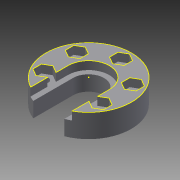
# Autodesk Inventor part: Kossel E3D V6 Mount
Saved by Autodesk Inventor 2013 (Build 170138000, 138)
## iProperties
Created: 2014-06-22
Part Number: Kossel E3D V6 Mount
Material: Generic
Document SubType Name: Modeling
Designer: Enlightx
Density: 1 g/cm^3
Author: Enlightx
Autodesk Inventor part; units mm, degrees
ref_plane "YZ Plane" through (0, 0, 0) normal (1, 0, 0) x (0, 1, 0)
ref_plane "XZ Plane" through (0, 0, 0) normal (0, 1, 0) x (-1, 0, 0)
ref_plane "XY Plane" through (0, 0, 0) normal (0, 0, 1) x (1, 0, 0)
sketch "Sketch1" plane through (0, 0, 0) normal (0, 0, 1) x (1, 0, 0)
  circle A0 centre (0, 0) radius 16.5
  dimension "d0" = 33
  constraints: 1 centre point, 1 coincident
  measures "d0" diameter of A0
extrude "Body" add sketch "Sketch1" along normal blind 9
sketch "Sketch2" plane through (0, 0, 9) normal (0, 0, 1) x (1, 0, 0)
  circle A0 centre (0, 0) radius 16.5 projected
  circle A1 centre (0, 0) radius 6
  line L0 (-6, 0) -> (-6, -15.3704)
  line L1 (6, 0) -> (6, -15.3704)
  arc A2 (-6, -15.3704) -> (6, -15.3704) centre (0, 0) ccw
  dimension "d3" = 12
  constraints: 6 point on circle, 4 end point, 2 centre point, 2 tangent, 1 coincident, 1 concentric, 1 parallel, 1 vertical
  measures "d3" diameter of A1
extrude "Main Cutout" cut sketch "Sketch2" against normal blind 9 contours L0 A1 L1 A0 | A1 picked at (0.2411, -12.9009)
sketch "Sketch4" plane through (0, 0, 9) normal (0, 0, 1) x (1, 0, 0)
  line L0 (6, 0) -> (6, -15.3704) projected
  arc A0 (6, -15.3704) -> (-6, -15.3704) centre (0, 0) ccw projected
  line L1 (-6, -15.3704) -> (-6, 0) projected
  arc A1 (6, 0) -> (-6, 0) centre (0, 0) ccw projected
  circle A2 centre (0, 0) radius 8
  line L2 (-8, 0) -> (-8, -14.4309)
  line L3 (8, 0) -> (8, -14.4309)
  arc A3 (-8, -14.4309) -> (8, -14.4309) centre (0, 0) ccw
  dimension "d7" = 16
  constraints: 6 point on circle, 4 end point, 2 centre point, 2 parallel, 2 tangent, 1 coincident, 1 concentric
  measures "d7" diameter of A2
extrude "Bottom Cutout" cut sketch "Sketch4" against normal blind 3.2 contours A1 L1 A2 L0 | A2 L3 A0 L0 | L1 A0 L2 A2 picked at (-6.3631, -2.9996)
sketch "Sketch7" plane through (0, 0, 0) normal (0, 0, -1) x (-1, 0, 0)
  arc A0 (6, 0) -> (-6, 0) centre (0, 0) ccw projected
  arc A1 (6, -15.3704) -> (-6, -15.3704) centre (0, 0) ccw projected
  circle A2 centre (0, 0) radius 12.5 construction
  circle A3 centre (0, 12.5) radius 1.6
  circle A4 centre (-10.8253, 6.25) radius 1.6
  circle A5 centre (-10.8253, -6.25) radius 1.6
  circle A6 centre (0, -12.5) radius 1.6
  circle A7 centre (10.8253, -6.25) radius 1.6
  circle A8 centre (10.8253, 6.25) radius 1.6
  dimension "d18" = 25
  dimension "d19" = 3.2
  dimension "d22" = 360
  constraints: 6 centre point, 1 coincident, 1 vertical alignment, 15 other
  measures "d19" diameter of A3
extrude "M3 Holes" cut sketch "Sketch7" against normal blind 7 contours A3 | A4 | A5 | A7 | A8
sketch "Sketch8" plane through (0, 0, 9) normal (0, 0, 1) x (1, 0, 0)
  arc A0 (8, 0) -> (-8, 0) centre (0, 0) ccw projected
  circle A1 centre (0, 0) radius 12.5 construction
  circle A2 centre (0, 12.5) radius 1.5 construction
  circle A3 centre (-10.8253, 6.25) radius 1.5 construction
  circle A4 centre (-10.8253, -6.25) radius 1.5 construction
  circle A5 centre (0, -12.5) radius 1.5 construction
  circle A6 centre (10.8253, -6.25) radius 1.5 construction
  circle A7 centre (10.8253, 6.25) radius 1.5 construction
  line L0 (0, 9.238) -> (-2.825, 10.869)
  line L1 (-2.825, 10.869) -> (-2.825, 14.131)
  line L2 (-2.825, 14.131) -> (0, 15.762)
  line L3 (0, 15.762) -> (2.825, 14.131)
  line L4 (2.825, 14.131) -> (2.825, 10.869)
  line L5 (2.825, 10.869) -> (0, 9.238)
  line L6 (-10.8253, 2.988) -> (-13.6503, 4.619)
  line L7 (-13.6503, 4.619) -> (-13.6503, 7.881)
  line L8 (-13.6503, 7.881) -> (-10.8253, 9.512)
  line L9 (-10.8253, 9.512) -> (-8.0003, 7.881)
  line L10 (-8.0003, 7.881) -> (-8.0003, 4.619)
  line L11 (-8.0003, 4.619) -> (-10.8253, 2.988)
  line L12 (10.8253, 2.988) -> (8.0003, 4.619)
  line L13 (8.0003, 4.619) -> (8.0003, 7.881)
  line L14 (8.0003, 7.881) -> (10.8253, 9.512)
  line L15 (10.8253, 9.512) -> (13.6503, 7.881)
  line L16 (13.6503, 7.881) -> (13.6503, 4.619)
  line L17 (13.6503, 4.619) -> (10.8253, 2.988)
  line L18 (-10.8253, -9.5178) -> (-13.6553, -7.8839)
  line L19 (-13.6553, -7.8839) -> (-13.6553, -4.6161)
  line L20 (-13.6553, -4.6161) -> (-10.8253, -2.9822)
  line L21 (-10.8253, -2.9822) -> (-7.9953, -4.6161)
  line L22 (-7.9953, -4.6161) -> (-7.9953, -7.8839)
  line L23 (-7.9953, -7.8839) -> (-10.8253, -9.5178)
  line L24 (10.8253, -9.5178) -> (7.9953, -7.8839)
  line L25 (7.9953, -7.8839) -> (7.9953, -4.6161)
  line L26 (7.9953, -4.6161) -> (10.8253, -2.9822)
  line L27 (10.8253, -2.9822) -> (13.6553, -4.6161)
  line L28 (13.6553, -4.6161) -> (13.6553, -7.8839)
  line L29 (13.6553, -7.8839) -> (10.8253, -9.5178)
  dimension "d26" = 25
  dimension "d27" = 3
  dimension "d30" = 360
  dimension "d32" = 5.65
  dimension "d33" = 5.65
  dimension "d34" = 5.65
  dimension "d35" = 5.66
  dimension "d36" = 5.66
  constraints: 60 end point, 6 centre point, 6 coincident, 1 vertical alignment, 80 other
  measures "d27" diameter of A2
  measures "d32" distance between parallel lines of L5 L2
  measures "d33" distance between parallel lines of L6 L9
  measures "d34" distance between parallel lines of L17 L14
  measures "d35" distance between parallel lines of L23 L20
  measures "d36" distance between parallel lines of L29 L26
extrude "M3 Nut Traps" cut sketch "Sketch8" against normal blind 3.2
sketch "Sketch9" plane through (0, 0, 9) normal (0, 0, 1) x (1, 0, 0)
  line L0 (-8, -7.8866) -> (-10.8253, -9.5178) projected
  line L1 (-10.8253, -9.5178) -> (-13.6553, -7.8839) projected
  line L2 (-13.6553, -7.8839) -> (-13.6553, -4.6161) projected
  line L3 (-13.6553, -4.6161) -> (-10.8253, -2.9822) projected
  line L4 (-10.8253, -2.9822) -> (-8, -4.6134) projected
  line L5 (-8, -4.6134) -> (-8, 0) projected
  arc A0 (8, 0) -> (-8, 0) centre (0, 0) ccw projected
  line L6 (8, 0) -> (8, -4.6134) projected
  line L7 (8, -4.6134) -> (10.8253, -2.9822) projected
  line L8 (10.8253, -2.9822) -> (13.6553, -4.6161) projected
  line L9 (13.6553, -4.6161) -> (13.6553, -7.8839) projected
  line L10 (13.6553, -7.8839) -> (10.8253, -9.5178) projected
  line L11 (10.8253, -9.5178) -> (8, -7.8866) projected
  line L12 (8, -7.8866) -> (8, -14.4309) projected
  arc A1 (8, -14.4309) -> (-8, -14.4309) centre (0, 0) ccw projected
  line L13 (-8, -14.4309) -> (-8, -7.8866) projected
  line L14 (13.6503, 4.619) -> (10.8253, 2.988) projected
  line L15 (10.8253, 2.988) -> (8.0003, 4.619) projected
  line L16 (8.0003, 4.619) -> (8.0003, 7.881) projected
  line L17 (8.0003, 7.881) -> (10.8253, 9.512) projected
  line L18 (10.8253, 9.512) -> (13.6503, 7.881) projected
  line L19 (13.6503, 7.881) -> (13.6503, 4.619) projected
  line L20 (2.825, 10.869) -> (0, 9.238) projected
  line L21 (0, 9.238) -> (-2.825, 10.869) projected
  line L22 (-2.825, 10.869) -> (-2.825, 14.131) projected
  line L23 (-2.825, 14.131) -> (0, 15.762) projected
  line L24 (0, 15.762) -> (2.825, 14.131) projected
  line L25 (2.825, 14.131) -> (2.825, 10.869) projected
  line L26 (-8.0003, 4.619) -> (-10.8253, 2.988) projected
  line L27 (-10.8253, 2.988) -> (-13.6503, 4.619) projected
  line L28 (-13.6503, 4.619) -> (-13.6503, 7.881) projected
  line L29 (-13.6503, 7.881) -> (-10.8253, 9.512) projected
  line L30 (-10.8253, 9.512) -> (-8.0003, 7.881) projected
  line L31 (-8.0003, 7.881) -> (-8.0003, 4.619) projected
body "Solid1"
